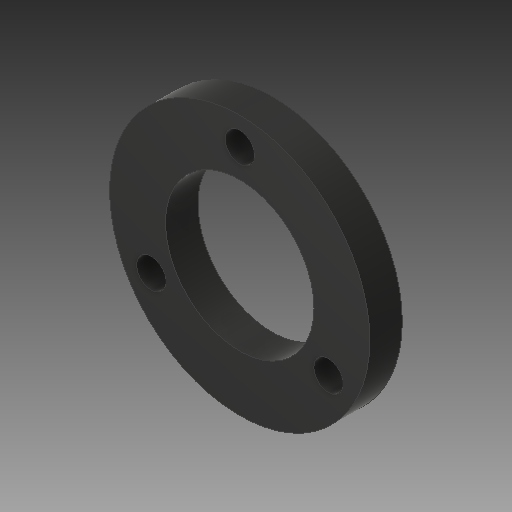
# Autodesk Inventor part: TA06
Saved by Autodesk Inventor 2017 (Build 210142000, 142)
## iProperties
Created: 2018-10-22
Part Number: TA06
Material: ABS Plastic
Document SubType Name: Modeling
Designer: Dell
Density: 1.06 g/cm^3
Appearance: Smooth - Black
Author: Dell
Autodesk Inventor part; units mm, degrees
ref_plane "YZ Plane" through (0, 0, 0) normal (1, 0, 0) x (0, 1, 0)
ref_plane "XZ Plane" through (0, 0, 0) normal (0, 1, 0) x (-1, 0, 0)
ref_plane "XY Plane" through (0, 0, 0) normal (0, 0, 1) x (1, 0, 0)
sketch "Sketch1" plane through (0, 0, 0) normal (0, 0, 1) x (1, 0, 0)
  circle A0 centre (0, 0) radius 12.7
  circle A1 centre (0, 0) radius 22.25
  circle A2 centre (0, 17.5) radius 2.5
  circle A3 centre (-15.1554, -8.75) radius 2.5
  circle A4 centre (15.1554, -8.75) radius 2.5
  dimension "d0" = 25.4
  dimension "d1" = 44.5
  dimension "d2" = 5
  dimension "d3" = 17.5
  dimension "d6" = 360
  constraints: 5 centre point, 2 coincident, 1 vertical alignment, 7 other
  measures "d0" diameter of A0
  measures "d1" diameter of A1
  measures "d2" diameter of A2
  measures "d3" distance of point (0, 0) A2.centre
extrude "Extrusion1" add sketch "Sketch1" along normal blind 5.55
body "Solid1"
